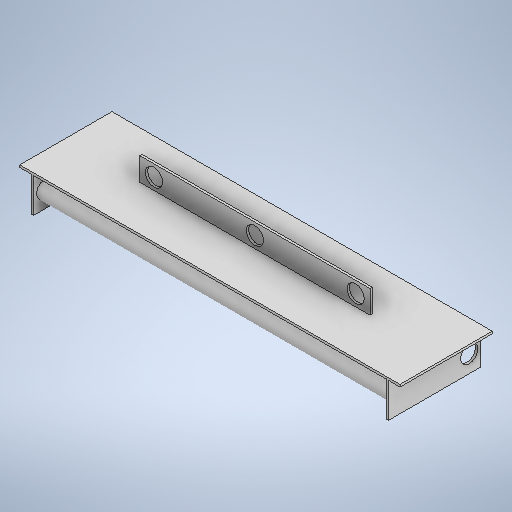
# Autodesk Inventor part: Claw_Platform_2
Saved by Autodesk Inventor 2025.2 (Build 292293000, 293)
## iProperties
Created: 2025-02-11
Part Number: Claw_Platform_2
Material: Generic
Document SubType Name: Modeling
Designer: Khushal
Density: 1 g/cm^3
Appearance: Default
Author: Khushal
Autodesk Inventor part; units mm, degrees
ref_plane "YZ Plane" through (0, 0, 0) normal (1, 0, 0) x (0, 1, 0)
ref_plane "XZ Plane" through (0, 0, 0) normal (0, 1, 0) x (-1, 0, 0)
ref_plane "XY Plane" through (0, 0, 0) normal (0, 0, 1) x (1, 0, 0)
sketch "Sketch1" plane through (0, 0, 0) normal (0, 0, 1) x (1, 0, 0)
  point P0 (0, 0)
sketch "Sketch2" plane through (0, 0, 0) normal (0, 1, 0) x (-1, 0, 0)
  line L0 (0, 0) -> (-330, 0)
  line L1 (-330, 0) -> (-330, 80)
  line L2 (-330, 80) -> (0, 80)
  line L3 (0, 80) -> (0, 0)
  dimension "d0" = 330
  dimension "d1" = 80
  constraints: 8 end point, 2 parallel, 1 horizontal, 1 perpendicular
  measures "d0" distance of L1.end L2.end
  measures "d1" distance of L0.end L1.end
extrude "Extrusion1" add sketch "Sketch2" along normal blind 2
sketch "Sketch3" plane through (0, 2, 0) normal (0, 1, 0) x (1, 0, 0)
  line L0 (0, 0) -> (0, -80) projected
  line L1 (330, -80) -> (330, 0) projected
  line L2 (0, -39) -> (0, -41)
  line L3 (330, -39) -> (330, -41)
  line L4 (165, -39) -> (65, -39)
  line L5 (65, -39) -> (65, -41)
  line L6 (65, -41) -> (265, -41)
  line L7 (265, -41) -> (265, -39)
  line L8 (165, -39) -> (265, -39)
  dimension "d5" = 165
  dimension "d6" = 100
  dimension "d7" = 2
  dimension "d8" = 200
  constraints: 14 end point, 4 point on line, 1 collinear, 1 parallel
  measures "d5" distance of L4.start L2.start
  measures "d6" distance of L4.start L4.end
  measures "d7" distance of L4.end L5.end
  measures "d8" distance of L5.end L6.end
extrude "Extrusion2" add sketch "Sketch3" along normal blind 20
sketch "Sketch4" plane through (65, 2, 41) normal (0, 0, 1) x (1, 0, 0)
  circle A0 centre (100, 10) radius 7.5
  circle A1 centre (12.5, 10) radius 7.5
  circle A2 centre (187.5, 10) radius 7.5
  point P0 (-65, -2)
  dimension "d11" = 15
  dimension "d12" = 15
  dimension "d13" = 15
  constraints: 3 centre point
  measures "d11" diameter of A0
  measures "d12" diameter of A1
  measures "d13" diameter of A2
extrude "Extrusion3" cut sketch "Sketch4" against normal through all
sketch "Sketch5" plane through (0, 0, 0) normal (0, -1, 0) x (1, 0, 0)
  line L0 (0, 80) -> (330, 80) projected
  line L1 (10, 0) -> (12, 0)
  line L2 (12, 0) -> (12, 80)
  line L3 (12, 80) -> (10, 80)
  line L4 (10, 80) -> (10, 0)
  line L5 (330, 0) -> (0, 0) projected
  line L6 (320, 0) -> (318, 0)
  line L7 (318, 0) -> (318, 80)
  line L8 (318, 80) -> (320, 80)
  line L9 (320, 80) -> (320, 0)
  dimension "d16" = 2
  dimension "d17" = 2
  constraints: 16 end point, 4 parallel, 3 point on line, 2 horizontal, 2 perpendicular
  measures "d16" distance of L3.end L2.end
  measures "d17" distance of L7.end L8.end
extrude "Extrusion4" add sketch "Sketch5" along normal blind 30 contours L0 L2 L1 L4 | L0 L9 L5 L7
sketch "Sketch6" plane through (10, 0, 0) normal (-1, 0, 0) x (0, 0, 1)
  circle A0 centre (70, -15) radius 7.5
  point P0 (0, 0)
  dimension "d23" = 15
  constraints: 1 centre point
  measures "d23" diameter of A0
extrude "Extrusion5" add sketch "Sketch6" against normal blind 310
sketch "Sketch7" plane through (10, 0, 0) normal (-1, 0, 0) x (0, 0, 1)
  circle A0 centre (10, -15) radius 7.5
  point P0 (0, 0)
  dimension "d26" = 15
  constraints: 1 centre point
  measures "d26" diameter of A0
extrude "Extrusion6" cut sketch "Sketch7" against normal through all
body "Solid1"
